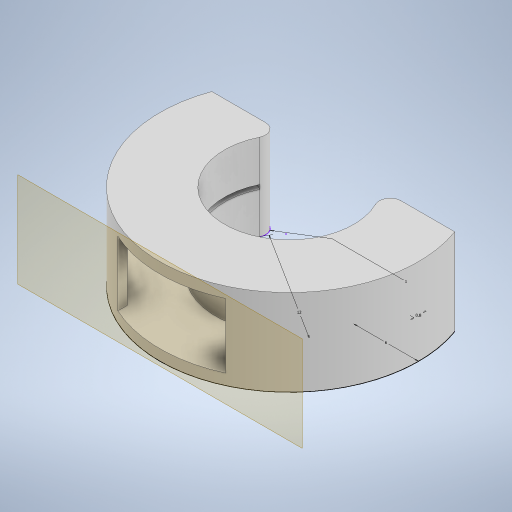
# Autodesk Inventor part: ir다이오드2
Saved by Autodesk Inventor 2023 (Build 270158000, 158)
## iProperties
Created: 2023-04-25
Part Number: ir다이오드2
Material: 일반
Document SubType Name: Modeling
Designer: rlatk
Density: 1 g/cm^3
Appearance: 기본값
Author: rlatk
Autodesk Inventor part; units mm, degrees
ref_plane "YZ Plane" through (0, 0, 0) normal (1, 0, 0) x (0, 1, 0)
ref_plane "XZ Plane" through (0, 0, 0) normal (0, 1, 0) x (-1, 0, 0)
ref_plane "XY Plane" through (0, 0, 0) normal (0, 0, 1) x (1, 0, 0)
sketch "스케치1" plane through (0, 0, 0) normal (0, 1, 0) x (-1, 0, 0)
  arc A0 (5.3819, -2.6523) -> (-5.3819, -2.6523) centre (0, 0) ccw
  arc A1 (11.2799, -4.0944) -> (-11.2799, -4.0944) centre (0, 0) ccw
  line L0 (11.2799, -4.0944) -> (6.2789, -4.0944)
  line L1 (-6.2789, -4.0944) -> (-11.2799, -4.0944)
  arc A2 (5.3819, -2.6523) -> (6.2789, -4.0944) centre (6.2789, -3.0944) ccw
  arc A3 (-6.2789, -4.0944) -> (-5.3819, -2.6523) centre (-6.2789, -3.0944) ccw
  arc A4 (10.7045, -3.2944) -> (-10.7045, -3.2944) centre (0, 0) ccw
  line L2 (10.7045, -3.2944) -> (6.2789, -3.2944)
  arc A5 (6.0995, -3.006) -> (6.2789, -3.2944) centre (6.2789, -3.0944) ccw
  arc A6 (6.0995, -3.006) -> (-6.0995, -3.006) centre (0, 0) ccw
  arc A7 (-6.2789, -3.2944) -> (-6.0995, -3.006) centre (-6.2789, -3.0944) ccw
  line L3 (-6.2789, -3.2944) -> (-10.7045, -3.2944)
  line L4 (-6.0995, -3.006) -> (-5.3819, -2.6523)
  line L5 (6.0995, -3.006) -> (5.3819, -2.6523)
  point P0 (-4.3859, -4.0944)
  point P1 (4.3859, -4.0944)
  dimension "d0" = 12
  dimension "d1" = 6
  dimension "d2" = 1
  dimension "d5" = 0.8
  constraints: 18 point on circle, 12 end point, 8 centre point, 4 tangent, 2 horizontal, 2 point on line, 1 coincident, 1 equal radius, 5 other
  measures "d0" diameter of A0
  measures "d1" radial gap between concentric circles of A0 A1
  measures "d2" radius of A2
  measures "d5" distance between parallel lines of L1 L3
extrude "돌출7" add sketch "스케치1" along normal blind 8
extrude "돌출8" cut sketch "스케치1" along normal blind 7 contours A6 A7 L3 A4 L2 A5
extrude "돌출9" add sketch "스케치1" along normal blind 1 contours A6 A7 L3 A4 L2 A5
extrude "돌출10" cut sketch "스케치1" along normal blind 4.2 contours A0 L4 A6 L5
extrude "돌출11" add sketch "스케치1" along normal blind 3.8 contours A0 L4 A6 L5
ref_plane "작업 평면2" through (0, 0, 12) normal (0, 0, 1) x (1, 0, 0)
sketch "스케치4" plane through (0, 0, 12) normal (0, 0, 1) x (1, 0, 0)
  line L0 (11.2, 7) -> (-11.2, 7) projected
  line L1 (-11.2, 1) -> (11.2, 1) projected
  line L2 (11.2, 1) -> (11.2, 7) projected
  line L3 (-11.2, 1) -> (-11.2, 7) projected
  line L4 (12, 8) -> (-12, 8) projected
  line L5 (12, 0) -> (-12, 0) projected
  line L6 (0, 7) -> (5, 7)
  line L7 (5, 7) -> (5, 1)
  line L8 (5, 1) -> (0, 1)
  line L9 (0, 7) -> (-5, 7)
  line L10 (-5, 7) -> (-5, 1)
  line L11 (-5, 1) -> (0, 1)
  line L12 (0, 8) -> (0, 7)
  line L13 (0, 1) -> (0, 0)
  point P0 (-10.7045, 7)
  point P1 (10.7045, 7)
  point P2 (10.7045, 1)
  point P3 (-10.7045, 1)
  point P4 (-11.2799, 8)
  point P5 (11.2799, 8)
  point P6 (-11.2799, 0)
  point P7 (11.2799, 0)
  dimension "d27" = 5
  constraints: 16 end point, 3 midpoint, 3 perpendicular, 2 point on line
  measures "d27" distance of L6.start L6.end
extrude "돌출12" cut sketch "스케치4" against normal blind 3.8 contours L7 L1 L10 L0
